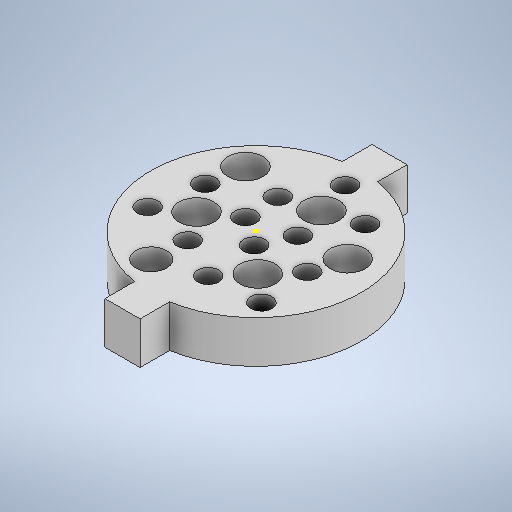
# Autodesk Inventor part: joy stick part 1
Saved by Autodesk Inventor 2025.2 (Build 292293000, 293)
## iProperties
Created: 2025-04-03
Part Number: joy stick part 1
Material: Generic
Document SubType Name: Modeling
Designer: avnr2
Density: 1 g/cm^3
Appearance: Default
Author: avnr2
Autodesk Inventor part; units mm, degrees
ref_plane "YZ Plane" through (0, 0, 0) normal (1, 0, 0) x (0, 1, 0)
ref_plane "XZ Plane" through (0, 0, 0) normal (0, 1, 0) x (-1, 0, 0)
ref_plane "XY Plane" through (0, 0, 0) normal (0, 0, 1) x (1, 0, 0)
sketch "Sketch1" plane through (0, 0, 0) normal (0, 1, 0) x (-1, 0, 0)
  circle A0 centre (0, 0) radius 15
  line L0 (0, -15) -> (0, -19)
  line L1 (0, -19) -> (2.5, -19)
  line L2 (2.5, -19) -> (2.5, -14.7902)
  line L3 (0, -19) -> (-2.5, -19)
  line L4 (-2.5, -19) -> (-2.5, -14.7902)
  line L5 (6.6169, 0) -> (-6.6879, 0)
  line L6 (0, 15) -> (0, 19)
  line L7 (0, 19) -> (2.5, 19)
  line L8 (2.5, 19) -> (2.5, 14.7902)
  line L9 (0, 19) -> (-2.5, 19)
  line L10 (-2.5, 19) -> (-2.5, 14.7902)
  point P0 (2.5, 14.7902)
  point P1 (-2.5, 14.7902)
  dimension "d0" = 4
  dimension "d1" = 2.5
  dimension "d13" = 30
  constraints: 22 end point, 8 symmetric about line, 2 perpendicular, 2 point on circle, 1 centre point, 1 coincident, 1 horizontal, 1 vertical
  measures "d0" distance of L0.start L0.end
  measures "d1" distance of L0.end L1.end
  measures "d13" diameter of A0
extrude "Extrusion1" add sketch "Sketch1" along normal blind 6
sketch "Sketch2" plane through (0, 6, 0) normal (0, 1, 0) x (1, 0, 0)
  circle A0 centre (2.0473, 7.2692) radius 2.5
  circle A1 centre (2.0473, 7.2692) radius 5 construction
  circle A2 centre (6.8395, 8.6957) radius 1.5
  circle A3 centre (2.0473, 7.2692) radius 5 construction
  circle A4 centre (0.6208, 12.0614) radius 1.5
  circle A5 centre (2.0473, 7.2692) radius 5 construction
  circle A6 centre (-2.7449, 5.8427) radius 1.5
  circle A7 centre (2.0473, 7.2692) radius 5 construction
  circle A8 centre (3.4738, 2.477) radius 1.5
  circle A9 centre (-6.6513, -1.8166) radius 2.5
  circle A10 centre (-6.6513, -1.8166) radius 5 construction
  circle A11 centre (-9.5082, 2.2868) radius 1.5
  circle A12 centre (-6.6513, -1.8166) radius 5 construction
  circle A13 centre (-10.7547, -4.6735) radius 1.5
  circle A14 centre (-6.6513, -1.8166) radius 5 construction
  circle A15 centre (-3.7944, -5.92) radius 1.5
  circle A16 centre (-6.6513, -1.8166) radius 5 construction
  circle A17 centre (-2.5478, 1.0403) radius 1.5
  circle A18 centre (5.3395, -5.0913) radius 2.5
  circle A19 centre (5.3395, -5.0913) radius 5 construction
  circle A20 centre (2.0648, -8.8697) radius 1.5
  circle A21 centre (5.3395, -5.0913) radius 5 construction
  circle A22 centre (9.1179, -8.3659) radius 1.5
  circle A23 centre (5.3395, -5.0913) radius 5 construction
  circle A24 centre (8.6142, -1.3128) radius 1.5
  circle A25 centre (5.3395, -5.0913) radius 5 construction
  circle A26 centre (1.5611, -1.8166) radius 1.5
  circle A27 centre (-8.7734, 7.2692) radius 2.5
  circle A28 centre (9.859, 3.1889) radius 2.5
  circle A29 centre (-4.0478, -10.8701) radius 2.1836
  dimension "d17" = 10
  dimension "d23" = 10
  dimension "d35" = 10
  dimension "d16" = 5
  dimension "d18" = 3
  dimension "d19" = 360
  dimension "d22" = 5
  dimension "d24" = 3
  dimension "d25" = 360
  dimension "d34" = 5
  dimension "d36" = 3
  dimension "d37" = 360
  dimension "d38" = 5
  dimension "d39" = 5
  constraints: 18 centre point, 12 coincident, 93 other
  measures "d16" diameter of A0
  measures "d18" diameter of A2
  measures "d22" diameter of A9
  measures "d24" diameter of A11
  measures "d34" diameter of A18
  measures "d36" diameter of A20
  measures "d38" diameter of A27
  measures "d39" diameter of A28
extrude "Extrusion2" cut sketch "Sketch2" against normal blind 5
sketch "Sketch3" plane through (0, 6, 0) normal (0, 1, 0) x (1, 0, 0)
  point P0 (0, 0)
body "Solid1"
